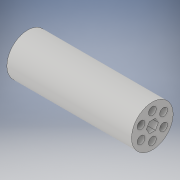
# Autodesk Inventor part: winch drum
Saved by Autodesk Inventor 2017 (Build 210142000, 142)
## iProperties
Created: 2017-01-27
Part Number: winch drum
Material: Generic
Document SubType Name: Modeling
Designer: Ben
Density: 1 g/cm^3
Appearance: Default
Author: Ben
Autodesk Inventor part; units mm, degrees
ref_plane "YZ Plane" through (0, 0, 0) normal (1, 0, 0) x (0, 1, 0)
ref_plane "XZ Plane" through (0, 0, 0) normal (0, 1, 0) x (-1, 0, 0)
ref_plane "XY Plane" through (0, 0, 0) normal (0, 0, 1) x (1, 0, 0)
sketch "Sketch1" plane through (0, 0, 0) normal (1, 0, 0) x (0, 1, 0)
  line L0 (0, -7.3323) -> (-6.35, -3.6662)
  line L1 (-6.35, -3.6662) -> (-6.35, 3.6662)
  line L2 (-6.35, 3.6662) -> (0, 7.3323)
  line L3 (0, 7.3323) -> (6.35, 3.6662)
  line L4 (6.35, 3.6662) -> (6.35, -3.6662)
  line L5 (6.35, -3.6662) -> (0, -7.3323)
  circle A0 centre (0, 0) radius 25.4
  line L6 (0, 0) -> (15.875, 0) construction
  circle A1 centre (15.875, 0) radius 4.7625
  circle A2 centre (7.9375, 13.7482) radius 4.7625
  line L7 (0, 0) -> (7.9375, 13.7482) construction
  circle A3 centre (-7.9375, 13.7482) radius 4.7625
  line L8 (0, 0) -> (-7.9375, 13.7482) construction
  circle A4 centre (-15.875, 0) radius 4.7625
  line L9 (0, 0) -> (-15.875, 0) construction
  circle A5 centre (-7.9375, -13.7482) radius 4.7625
  line L10 (0, 0) -> (-7.9375, -13.7482) construction
  circle A6 centre (7.9375, -13.7482) radius 4.7625
  line L11 (0, 0) -> (7.9375, -13.7482) construction
  dimension "d0" = 12.7
  dimension "d1" = 50.8
  dimension "d2" = 9.525
  dimension "d3" = 15.875
  dimension "d6" = 360
  constraints: 24 end point, 9 coincident, 7 centre point, 1 horizontal, 1 vertical, 44 other
  measures "d0" distance between parallel lines of L1 L4
  measures "d1" diameter of A0
  measures "d2" diameter of A1
  measures "d3" distance of L6.start L6.end
extrude "Extrusion1" add sketch "Sketch1" along normal blind 152.4
body "Solid1"
